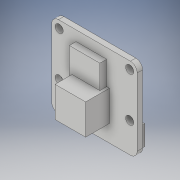
# Autodesk Inventor part: RasPIcam
Saved by Autodesk Inventor 2019 (Build 230136000, 136)
## iProperties
Created: 2019-02-12
Part Number: RasPIcam
Material: Generic
Document SubType Name: Modeling
Designer: izsoandras
Density: 1 g/cm^3
Appearance: Default
Author: izsoandras
Autodesk Inventor part; units mm, degrees
ref_plane "YZ Plane" through (0, 0, 0) normal (1, 0, 0) x (0, 1, 0)
ref_plane "XZ Plane" through (0, 0, 0) normal (0, 1, 0) x (-1, 0, 0)
ref_plane "XY Plane" through (0, 0, 0) normal (0, 0, 1) x (1, 0, 0)
sketch "Sketch2" plane through (0, 0, 0) normal (0, 0, 1) x (1, 0, 0)
  line L0 (-10.0737, 8.3897) -> (11.1263, 8.3897)
  line L1 (13.1263, 6.3897) -> (13.1263, -13.6103)
  line L2 (11.1263, -15.6103) -> (-10.0737, -15.6103)
  line L3 (-12.0737, -13.6103) -> (-12.0737, 6.3897)
  arc A0 (-10.0737, 8.3897) -> (-12.0737, 6.3897) centre (-10.0737, 6.3897) ccw
  arc A1 (13.1263, 6.3897) -> (11.1263, 8.3897) centre (11.1263, 6.3897) ccw
  arc A2 (11.1263, -15.6103) -> (13.1263, -13.6103) centre (11.1263, -13.6103) ccw
  arc A3 (-12.0737, -13.6103) -> (-10.0737, -15.6103) centre (-10.0737, -13.6103) ccw
  point P0 (0, 0)
  point P1 (-12.0737, 8.3897)
  point P2 (13.1263, -15.6103)
  point P3 (13.1263, 8.3897)
  point P4 (-12.0737, -15.6103)
  dimension "d0" = 25.2
  dimension "d1" = 24
  dimension "d4" = 2
  constraints: 8 end point, 8 point on circle, 8 point on line, 8 tangent, 4 centre point, 3 equal radius, 2 parallel, 1 horizontal, 1 perpendicular
  measures "d0" distance of point (-12.074, 8.39) point (13.126, 8.39)
  measures "d1" distance of point (-12.074, -15.61) point (-12.074, 8.39)
  measures "d4" radius of A0
extrude "Extrusion1" add sketch "Sketch2" along normal blind 1.6
sketch "Sketch3" plane through (0, 0, 1.6) normal (0, 0, 1) x (1, 0, 0)
  circle A0 centre (-9.8737, 6.1897) radius 1.2
  circle A1 centre (10.9263, 6.1897) radius 1.2
  circle A2 centre (10.9263, -6.8103) radius 1.2
  circle A3 centre (-9.8737, -6.8103) radius 1.2
  line L0 (11.1263, 8.3897) -> (-10.0737, 8.3897) projected
  line L1 (-12.0737, 6.3897) -> (-12.0737, -13.6103) projected
  line L2 (13.1263, -13.6103) -> (13.1263, 6.3897) projected
  point P0 (0, 0)
  dimension "d5" = 2.4
  dimension "d6" = 2.4
  dimension "d7" = 2.4
  dimension "d8" = 2.4
  dimension "d9" = 2.2
  dimension "d10" = 2.2
  dimension "d11" = 2.2
  dimension "d12" = 2.2
  dimension "d13" = 2.2
  dimension "d14" = 2.2
  dimension "d15" = 13
  dimension "d16" = 13
  constraints: 4 centre point
  measures "d5" diameter of A0
  measures "d6" diameter of A1
  measures "d7" diameter of A2
  measures "d8" diameter of A3
  measures "d9" distance from line of L0 A0.centre
  measures "d10" distance from line of L1 A0.centre
  measures "d11" distance from line of L0 A1.centre
  measures "d12" distance from line of L2 A1.centre
  measures "d13" distance from line of L1 A3.centre
  measures "d14" horizontal distance of L2.start A2.centre
  measures "d15" distance of A3.centre A0.centre
  measures "d16" distance of A1.centre A2.centre
extrude "Extrusion2" cut sketch "Sketch3" against normal up to next
sketch "Sketch4" plane through (0, 0, 1.6) normal (0, 0, 1) x (1, 0, 0)
  line L0 (-4.8737, 5.3897) -> (4.1263, 5.3897)
  line L1 (4.1263, 5.3897) -> (4.1263, -2.6103)
  line L2 (4.1263, -2.6103) -> (-4.8737, -2.6103)
  line L3 (-4.8737, -2.6103) -> (-4.8737, 5.3897)
  line L4 (11.1263, 8.3897) -> (-10.0737, 8.3897) projected
  line L5 (13.1263, -13.6103) -> (13.1263, 6.3897) projected
  point P0 (0, 0)
  dimension "d19" = 9
  dimension "d20" = 8
  dimension "d21" = 3
  dimension "d22" = 9
  constraints: 8 end point, 2 parallel, 1 horizontal, 1 perpendicular
  measures "d19" distance of L0.start L0.end
  measures "d20" distance of L0.end L1.end
  measures "d21" distance between parallel lines of L4 L0
  measures "d22" distance between parallel lines of L5 L1
extrude "Extrusion3" add sketch "Sketch4" along normal blind 2
sketch "Sketch5" plane through (0, 0, 1.6) normal (0, 0, 1) x (1, 0, 0)
  line L0 (-4.0737, -1.6103) -> (4.9263, -1.6103)
  line L1 (4.9263, -1.6103) -> (4.9263, -10.6103)
  line L2 (4.9263, -10.6103) -> (-4.0737, -10.6103)
  line L3 (-4.0737, -10.6103) -> (-4.0737, -1.6103)
  line L4 (-10.0737, -15.6103) -> (11.1263, -15.6103) projected
  line L5 (-12.0737, 6.3897) -> (-12.0737, -13.6103) projected
  point P0 (0, 0)
  dimension "d25" = 9
  dimension "d26" = 9
  dimension "d27" = 5
  dimension "d28" = 8
  constraints: 8 end point, 2 parallel, 1 horizontal, 1 perpendicular
  measures "d25" distance of L0.start L0.end
  measures "d26" distance of L2.end L0.start
  measures "d27" distance between parallel lines of L4 L2
  measures "d28" distance between parallel lines of L5 L3
extrude "Extrusion4" add sketch "Sketch5" along normal blind 7
sketch "Sketch6" plane through (0, 0, 0) normal (0, 0, -1) x (-1, 0, 0)
  line L0 (10.0737, -15.6103) -> (-11.1263, -15.6103) projected
  line L1 (-11.0263, -15.6103) -> (9.9737, -15.6103)
  line L2 (9.9737, -15.6103) -> (9.9737, -9.8103)
  line L3 (9.9737, -9.8103) -> (-11.0263, -9.8103)
  line L4 (-11.0263, -9.8103) -> (-11.0263, -15.6103)
  line L5 (-13.1263, 6.3897) -> (-13.1263, -13.6103) projected
  point P0 (0, 0)
  dimension "d31" = 21
  dimension "d32" = 5.8
  dimension "d33" = 2.1
  constraints: 8 end point, 2 parallel, 1 horizontal, 1 perpendicular, 1 point on line
  measures "d31" distance of L2.end L3.end
  measures "d32" distance of L3.end L1.start
  measures "d33" distance between parallel lines of L5 L4
extrude "Extrusion5" add sketch "Sketch6" along normal blind 2.78
equation "\"d6\" = d5"
equation "\"d7\" = d5"
equation "\"d8\" = d5"
equation "\"d10\" = d9"
equation "\"d11\" = d9"
equation "\"d12\" = d9"
equation "\"d13\" = d9"
equation "\"d14\" = d9"
equation "\"d16\" = d15"
equation "\"d33\" = -0.5 * d31 + 0.5 * d0"
body "Solid1"
